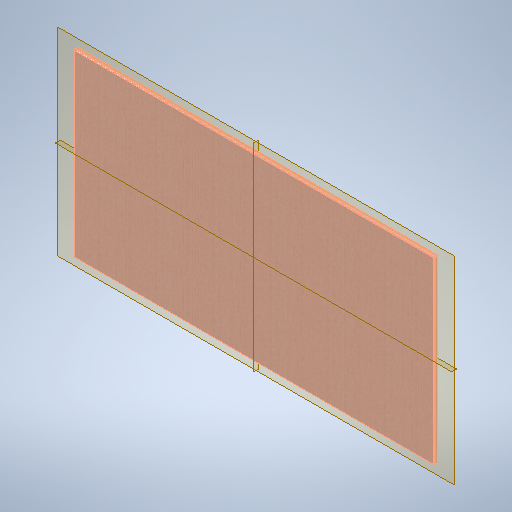
# Autodesk Inventor part: Tampo
Saved by Autodesk Inventor 2025.2 (Build 292293000, 293)
## iProperties
Created: 2025-04-02
Part Number: Tampo
Material: Wood (Oak)
Document SubType Name: Modeling
Designer: kenne
Density: 0.76 g/cm^3
Appearance: White Oak - Natural Medium Gloss
Author: kenne
Autodesk Inventor part; units mm, degrees
sketch "Tampo_sketch" plane through (0, 0, 0) normal (0, 0, 1) x (1, 0, 0)
  line L0 (-800, 400) -> (800, 400)
  line L1 (800, 400) -> (800, -400)
  line L2 (800, -400) -> (-800, -400)
  line L3 (-800, -400) -> (-800, 400)
  line L4 (-800, 400) -> (800, -400) construction
  line L5 (800, 400) -> (-800, -400) construction
  point P0 (0, 0)
  point P1 (0, 0)
  dimension "d0" = 1600
  dimension "d1" = 800
  constraints: 12 end point, 2 midpoint, 2 parallel, 1 coincident, 1 horizontal, 1 perpendicular
  measures "d0" distance of L0.start L0.end
  measures "d1" distance of L2.end L0.start
extrude "Tampo_Extrusion" add sketch "Tampo_sketch" along normal mid plane 20
fillet "Fillet1" radius 3 12 edges at (800, 400, 0) (-800, 400, 0) (-800, -400, 0) (800, -400, 0) (0, -400, 10) (0, -400, -10) (800, 0, 10) (800, 0, -10) (-800, 0, 10) (-800, 0, -10) (0, 400, 10) (0, 400, -10)
